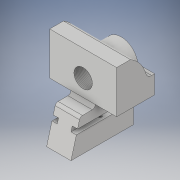
# Autodesk Inventor part: VS-002 (SLIDING JAW)
Saved by Autodesk Inventor 2017 SP1 (Build 210196100, 196)
## iProperties
Created: 2016-11-30
Part Number: VS-002 (SLIDING JAW)
Material: Generic
Document SubType Name: Modeling
Designer: OCCC
Density: 1 g/cm^3
Appearance: Default
Author: OCCC
Autodesk Inventor part; units mm, degrees
ref_plane "YZ Plane" through (0, 0, 0) normal (1, 0, 0) x (0, 1, 0)
ref_plane "XZ Plane" through (0, 0, 0) normal (0, 1, 0) x (-1, 0, 0)
ref_plane "XY Plane" through (0, 0, 0) normal (0, 0, 1) x (1, 0, 0)
sketch "Sketch1" plane through (0, 0, 0) normal (1, 0, 0) x (0, 1, 0)
  line L0 (0, 0) -> (44.45, 0)
  line L1 (44.45, 0) -> (44.45, -14.4312)
  arc A0 (23.6904, -30.4604) -> (44.45, -14.4312) centre (14.2875, 3.175) ccw
  line L2 (19.05, -36.5759) -> (19.05, -39.6875)
  line L3 (19.05, -39.6875) -> (0, -39.6875)
  line L4 (0, -39.6875) -> (0, 0)
  arc A1 (23.6904, -30.4604) -> (19.05, -36.5759) centre (25.4, -36.5759) ccw
  point P0 (19.05, -31.4238)
  dimension "d0" = 44.45
  dimension "d1" = 19.05
  dimension "d2" = 39.6875
  dimension "d3" = 30.1625
  dimension "d5" = 3.175
  dimension "d6" = 34.925
  dimension "d7" = 6.35
  constraints: 10 end point, 5 point on circle, 3 perpendicular, 2 centre point, 2 tangent, 1 horizontal, 1 point on line, 1 vertical
  measures "d0" distance of L0.start L0.end
  measures "d1" distance of L2.end L3.end
  measures "d2" distance of L3.end L0.start
  measures "d3" distance from line of L1 A0.centre
  measures "d5" distance from line of L0 A0.centre
  measures "d6" radius of A0
  measures "d7" radius of A1
extrude "Extrusion1" add sketch "Sketch1" along normal mid plane 69.85
sketch "Sketch2" plane through (34.925, 19.05, -39.6875) normal (0, 0, -1) x (-1, 0, 0)
  line L0 (0, 25.4) -> (0, -19.05) projected
  line L1 (0, 0) -> (0, -19.05)
  line L2 (69.85, 0) -> (69.85, -19.05) projected
  line L3 (0, 0) -> (69.85, 0) projected
  line L4 (69.85, -19.05) -> (69.85, 0)
  line L5 (34.925, -19.05) -> (34.925, -1.5875) construction
  arc A0 (52.3152, 0) -> (17.5348, 0) centre (34.925, -1.5875) ccw
  line L6 (69.85, -19.05) -> (0, -19.05) projected
  line L7 (22.225, -19.05) -> (22.225, -31.8897)
  line L8 (22.225, -31.8897) -> (27.7495, -31.8897)
  line L9 (27.7495, -31.8897) -> (27.7495, -36.6522)
  line L10 (27.7495, -36.6522) -> (22.225, -36.6522)
  line L11 (22.225, -36.6522) -> (22.225, -57.15)
  line L12 (22.225, -57.15) -> (47.625, -57.15)
  line L13 (47.625, -57.15) -> (47.625, -36.6522)
  line L14 (47.625, -36.6522) -> (42.1005, -36.6522)
  line L15 (42.1005, -36.6522) -> (42.1005, -31.8897)
  line L16 (42.1005, -31.8897) -> (47.625, -31.8897)
  line L17 (47.625, -31.8897) -> (47.625, -19.05)
  line L18 (0, -19.05) -> (22.225, -19.05)
  line L19 (47.625, -19.05) -> (69.85, -19.05)
  line L20 (69.85, 0) -> (52.3152, 0)
  line L21 (17.5348, 0) -> (0, 0)
  dimension "d10" = 34.925
  dimension "d11" = 22.225
  dimension "d13" = 55.5625
  dimension "d16" = 22.225
  dimension "d17" = 38.1
  dimension "d18" = 5.5245
  dimension "d19" = 4.7625
  dimension "d20" = 12.8397
  constraints: 36 end point, 16 perpendicular, 6 collinear, 6 point on line, 2 point on circle, 1 centre point, 1 coincident
  measures "d10" diameter of A0
  measures "d11" distance between parallel lines of L7 L0
  measures "d13" distance from line of L12 L5.end
  measures "d16" distance between parallel lines of L2 L17
  measures "d17" distance between parallel lines of L12 L19
  measures "d18" distance between parallel lines of L13 L15
  measures "d19" distance between parallel lines of L14 L16
  measures "d20" distance between parallel lines of L19 L16
extrude "Extrusion2" add sketch "Sketch2" against normal blind 65.0875
sketch "Sketch3" plane through (34.925, 0, 0) normal (1, 0, 0) x (0, 0, -1)
  line L0 (0, 0) -> (-25.4, 0)
  line L1 (-25.4, 0) -> (-25.4, 44.45)
  line L2 (-25.4, 44.45) -> (0, 44.45)
  line L3 (0, 44.45) -> (0, 0)
  dimension "d23" = 44.45
  dimension "d24" = 25.4
  constraints: 8 end point, 2 parallel, 1 horizontal, 1 perpendicular
  measures "d23" distance of L0.end L1.end
  measures "d24" distance of L1.end L2.end
extrude "Extrusion3" cut sketch "Sketch3" against normal blind 69.85
sketch "Sketch5" plane through (34.925, 0, 0) normal (1, 0, 0) x (0, 0, -1)
  line L0 (39.6875, -38.1) -> (-25.4, -38.1) projected
  line L1 (-25.4, 0) -> (-25.4, -12.8397) projected
  line L2 (-25.4, -38.1) -> (-25.4, 0)
  line L3 (39.6875, 0) -> (0, 0) projected
  line L4 (-25.4, 0) -> (0, 0)
  line L5 (0, 0) -> (0, 0)
  line L6 (-3.175, -3.175) -> (-13.4499, -3.175)
  line L7 (-16.5131, -5.5146) -> (-25.4, -38.1)
  arc A0 (-3.175, -3.175) -> (0, 0) centre (-3.175, 0) ccw
  arc A1 (-13.4499, -3.175) -> (-16.5131, -5.5146) centre (-13.4499, -6.35) ccw
  point P0 (-15.875, -3.175)
  dimension "d27" = 34.925
  dimension "d28" = 9.525
  dimension "d29" = 3.175
  dimension "d30" = 3.175
  constraints: 10 end point, 4 point on circle, 4 tangent, 3 perpendicular, 2 centre point, 2 point on line, 1 collinear
  measures "d27" vertical distance of L0.end point (-15.875, -3.175)
  measures "d28" distance from line of point (-15.875, -3.175) L1
  measures "d29" radius of A0
  measures "d30" radius of A1
extrude "Extrusion4" cut sketch "Sketch5" against normal blind 69.85
hole "Hole1" at (-7.9375, -38.1, -9.5123) direction (0, 1, 0) diameter 3.7973 depth 26.9875
hole "Hole2" at (7.9375, -38.1, -9.525) direction (0, 1, 0) diameter 3.7973 depth 26.9875
hole "Hole3" at (7.9375, -38.1, -9.525) direction (0, 1, 0) diameter 4.3434 depth 19.05 counterbore diameter 5.5563 counterbore depth 9.525 thread size "12-24 UNC" class "2B" standard "ANSI Unified Screw Threads"
hole "Hole4" at (-7.9375, -38.1, -9.5123) direction (0, 1, 0) diameter 4.3434 depth 19.05 counterbore diameter 5.5563 counterbore depth 9.525 thread size "12-24 UNC" class "2B" standard "ANSI Unified Screw Threads"
hole "Hole5" at (0, 17.4625, -39.6875) direction (0, 0, 1) diameter 19.2532 end through all thread size "13/16-20 UNEF" class "3B" standard "ANSI Unified Screw Threads"
body "Solid1"
